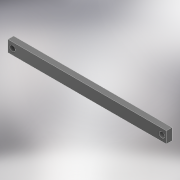
# Autodesk Inventor part: 3
Saved by Autodesk Inventor 2022 (Build 260153000, 153)
## iProperties
Created: 2023-12-24
Part Number: 3
Material: PMMA-Kunststoff
Document SubType Name: Modeling
Designer: alsaa
Density: 1.188 g/cm^3
Appearance: Glatt - Schwarz
Author: alsaa
## iProperties of the stored document 3_3D-Druck.ipt
Created: 2023-12-24
Part Number: 3_3D-Druck
Material: Generisch
Document SubType Name: Modeling
Designer: alsaa
Density: 1 g/cm^3
Appearance: Vorgabe
Author: alsaa
Autodesk Inventor part; units mm, degrees
ref_plane "YZ Plane" through (0, 0, 0) normal (1, 0, 0) x (0, 1, 0)
ref_plane "XZ Plane" through (0, 0, 0) normal (0, 1, 0) x (-1, 0, 0)
ref_plane "XY Plane" through (0, 0, 0) normal (0, 0, 1) x (1, 0, 0)
sketch "Skizze1" plane through (0, 0, 0) normal (0, 0, 1) x (1, 0, 0)
  line L0 (-53, -3.85) -> (53, -3.85)
  line L1 (53, -3.85) -> (53, 3.85)
  line L2 (53, 3.85) -> (-53, 3.85)
  line L3 (-53, 3.85) -> (-53, -3.85)
  line L4 (-53, -3.85) -> (53, 3.85) construction
  line L5 (53, -3.85) -> (-53, 3.85) construction
  point P0 (0, 0)
  dimension "d0" = 7.7
  dimension "d1" = 106
  constraints: 12 end point, 2 midpoint, 2 parallel, 1 horizontal, 1 perpendicular
  measures "d0" distance of L0.end L1.end
  measures "d1" distance of L1.end L2.end
extrude "Extrusion1" add sketch "Skizze1" along normal blind 3.8
sketch "Skizze2" plane through (0, 0, 3.8) normal (0, 0, 1) x (1, 0, 0)
  line L0 (53, 3.85) -> (-53, 3.85) construction
  line L1 (50, 3.85) -> (50, -3.85) construction
  line L2 (-53, -3.85) -> (53, -3.85) construction
  line L3 (53, -3.85) -> (53, 3.85) construction
  circle A0 centre (50, 0) radius 1.85
  line L4 (0, 3.85) -> (0, -3.85) construction
  circle A1 centre (-50, 0) radius 1.85
  point P0 (0, 0)
  dimension "d4" = 3
  dimension "d5" = 3.7
  constraints: 4 end point, 3 midpoint, 2 centre point, 2 point on line, 1 symmetric about line, 1 vertical, 1 other
  measures "d4" distance between parallel lines of L3 L1
  measures "d5" diameter of A0
extrude "Extrusion2" cut sketch "Skizze2" against normal through all
